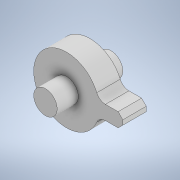
# Autodesk Inventor part: 2번부품
Saved by Autodesk Inventor 2022 (Build 260153000, 153)
## iProperties
Created: 2021-09-05
Part Number: 2번부품
Material: 일반
Document SubType Name: Modeling
Designer: 서울공업고등학교
Density: 1 g/cm^3
Appearance: 기본값
Author: 서울공업고등학교
Autodesk Inventor part; units mm, degrees
ref_plane "YZ Plane" through (0, 0, 0) normal (1, 0, 0) x (0, 1, 0)
ref_plane "XZ Plane" through (0, 0, 0) normal (0, 1, 0) x (-1, 0, 0)
ref_plane "XY Plane" through (0, 0, 0) normal (0, 0, 1) x (1, 0, 0)
sketch "스케치1" plane through (0, 0, 0) normal (0, 0, 1) x (1, 0, 0)
  circle A0 centre (0, 0) radius 2.5
  arc A1 (6.8374, 1.5) -> (6.8374, -1.5) centre (0, 0) ccw
  line L0 (6.8374, 1.5) -> (12, 1.5)
  line L1 (6.8374, -1.5) -> (12, -1.5)
  line L2 (12, 1.5) -> (12, -1.5)
  dimension "d0" = 5
  dimension "d1" = 14
  dimension "d2" = 3
  dimension "d3" = 1.5
  dimension "d4" = 12
  constraints: 6 end point, 2 centre point, 2 coincident, 2 horizontal, 2 point on circle, 1 perpendicular
  measures "d0" diameter of A0
  measures "d1" diameter of A1
  measures "d2" distance between parallel lines of L1 L0
  measures "d3" distance from line of point (0, 0) L0
  measures "d4" distance from line of point (0, 0) L2
extrude "돌출1" add sketch "스케치1" along normal mid plane 5
extrude "돌출2" add sketch "스케치1" along normal mid plane 14 contours A0
chamfer "모따기1" distance 1 angle 45 2 edges at (12, 1.5, 0) (12, -1.5, 0)
fillet "모깎기1" radius 2 2 edges at (6.8374, 1.5, 0) (6.8374, -1.5, 0)
